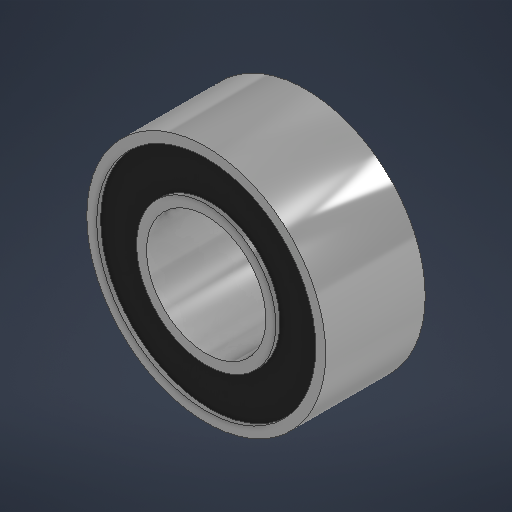
# Autodesk Inventor part: Miniatur Kugellager MR 63 2RS 3x6x2.5 mm
Saved by Autodesk Inventor 2026.1 (Build 301233020, 233B)
## iProperties
Created: 2025-12-14
Part Number: Miniatur Kugellager MR 63 2RS 3x6x2.5 mm
Material: Generic
Document SubType Name: Modeling
Designer: Bahaa
Density: 1 g/cm^3
Appearance: Default
Author: Bahaa
Autodesk Inventor part; units mm, degrees
ref_plane "YZ Plane" through (0, 0, 0) normal (1, 0, 0) x (0, 1, 0)
ref_plane "XZ Plane" through (0, 0, 0) normal (0, 1, 0) x (-1, 0, 0)
ref_plane "XY Plane" through (0, 0, 0) normal (0, 0, 1) x (1, 0, 0)
sketch "Sketch1" plane through (0, 0, 0) normal (0, 1, 0) x (-1, 0, 0)
  circle A0 centre (0, 0) radius 3
  circle A1 centre (0, 0) radius 1.5
  circle A2 centre (0, 0) radius 1.75
  circle A3 centre (0, 0) radius 2.75
  dimension "d0" = 6
  dimension "d1" = 3
  dimension "d2" = 3.5
  dimension "d3" = 5.5
  constraints: 4 centre point, 4 coincident
  measures "d0" diameter of A0
  measures "d1" diameter of A1
  measures "d2" diameter of A2
  measures "d3" diameter of A3
extrude "Extrusion1" add sketch "Sketch1" along normal blind 2.5 contours A0 | A2 | A3
extrude "Extrusion2" cut sketch "Sketch1" against normal blind 0.1 from surface at 2.5 contours A3
extrude "Extrusion3" cut sketch "Sketch1" along normal blind 0.1 contours A3
body "Solid1"
